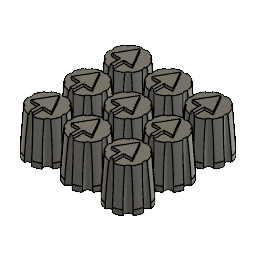
PotiKnobV3 (Autodesk Fusion 360 design; units mm, degrees)
Autodesk Fusion 360 part; units mm, degrees
sketch "Sketch1" plane through (0, 0, 0) normal (0, 1, 0) x (1, 0, 0)
  circle A0 centre (0, 0) radius 3.025
  circle A1 centre (0, 0) radius 7.5
  dimension "d1" = 6.05
  dimension "d2" = 15
  constraint coincident A0.centre A1.centre
  measures "d1" diameter of A0
  measures "d2" diameter of A1
extrude "Extrude1" add sketch "Sketch1" along normal blind 16 contours A0 | A1 makes body 1
extrude "Extrude2" cut sketch "Sketch1" along normal blind 12 contours A0 bodies 1
chamfer "Chamfer1" distance 1 distance2 3 1 edges at (-2.8203, 0, 1.0939) measured on face at (5.9804, 0, 0.3726) on bodies 1
sketch "Sketch2" plane through (0, 16, 0) normal (0, 1, 0) x (-1, 0, 0)
  circle A0 centre (0, 0) radius 7.5
  line L0 (0, 0) -> (0, -9.5957) construction
  circle A1 centre (0, -7.5) radius 1.3779
  circle A2 centre (5.3033, -5.3033) radius 1.3779
  circle A3 centre (7.5, 0) radius 1.3779
  circle A4 centre (5.3033, 5.3033) radius 1.3779
  circle A5 centre (0, 7.5) radius 1.3779
  circle A6 centre (-5.3033, 5.3033) radius 1.3779
  circle A7 centre (-7.5, 0) radius 1.3779
  circle A8 centre (-5.3033, -5.3033) radius 1.3779
  dimension "d10" = 360
  constraint coincident A0.centre L0.start
  constraint vertical L0
  constraint coincident L0 A1.centre
  constraint coincident A0 A1.centre
chamfer "Chamfer2" distance 1 distance2 14 1 edges at (-6.9925, 16, 2.7121) measured on face at (1.9158, 16, -2.8099) on bodies 1
extrude "Extrude3" cut sketch "Sketch2" against normal blind 17 contours A0 A3 | A0 A4 | A0 A2 | A0 A5 | A0 A1 | A0 A6 | A0 A8 | A0 A7 picked at (7.0559, -0.2871) picked at (4.9719, 4.9719) picked at (4.9719, -4.9719) picked at (0, 7.0313) picked at (0, -7.0313) picked at (-4.9932, 4.9519) picked at (-4.9932, -4.9519) picked at (-7.0313, 0) bodies 1
sketch "Sketch3" plane through (0, 16, 0) normal (0, 1, 0) x (-1, 0, 0)
  arc A0 (-3.9313, -5.1764) -> (-5.1764, -3.9313) centre (-5.3033, -5.3033) ccw
  arc A1 (-3.9313, -5.1764) -> (-0.8804, -6.4401) centre (0, 0) ccw
  arc A2 (0.8804, -6.4401) -> (-0.8804, -6.4401) centre (0, -7.5) ccw
  arc A3 (0.8804, -6.4401) -> (3.9313, -5.1764) centre (0, 0) ccw
  arc A4 (5.1764, -3.9313) -> (3.9313, -5.1764) centre (5.3033, -5.3033) ccw
  arc A5 (5.1764, -3.9313) -> (6.4401, -0.8804) centre (0, 0) ccw
  arc A6 (6.4401, 0.8804) -> (6.4401, -0.8804) centre (7.5, 0) ccw
  arc A7 (6.4401, 0.8804) -> (5.1764, 3.9313) centre (0, 0) ccw
  arc A8 (3.9313, 5.1764) -> (5.1764, 3.9313) centre (5.3033, 5.3033) ccw
  arc A9 (3.9313, 5.1764) -> (0.8804, 6.4401) centre (0, 0) ccw
  arc A10 (-0.8804, 6.4401) -> (0.8804, 6.4401) centre (0, 7.5) ccw
  arc A11 (-0.8804, 6.4401) -> (-3.9313, 5.1764) centre (0, 0) ccw
  arc A12 (-5.1764, 3.9313) -> (-3.9313, 5.1764) centre (-5.3033, 5.3033) ccw
  arc A13 (-5.1764, 3.9313) -> (-6.4401, 0.8804) centre (0, 0) ccw
  arc A14 (-6.4401, -0.8804) -> (-6.4401, 0.8804) centre (-7.5, 0) ccw
  arc A15 (-6.4401, -0.8804) -> (-5.1764, -3.9313) centre (0, 0) ccw
  line L0 (-4.0258, 2.3243) -> (0, -4.6486)
  line L1 (0, -4.6486) -> (4.0258, 2.3243)
  line L2 (4.0258, 2.3243) -> (-4.0258, 2.3243)
  line L3 (-0.6079, 6.7078) -> (0.6079, 6.7078)
  line L4 (0.6079, 6.7078) -> (0.6079, -6.7078)
  line L5 (0.6079, -6.7078) -> (-0.6079, -6.7078)
  line L6 (-0.6079, -6.7078) -> (-0.6079, 6.7078)
  line L7 (-0.6079, 6.7078) -> (0.6079, -6.7078) construction
  line L8 (0.6079, 6.7078) -> (-0.6079, -6.7078) construction
  constraint coincident A1.centre A3.centre
  constraint perpendicular L3 L4
  constraint parallel L3 L5
  constraint parallel L4 L6
  constraint horizontal L3
  constraint coincident L7 A1.centre
  constraint coincident L8 A1.centre
extrude "Extrude4" add sketch "Sketch3" along normal blind 1 contours L0 L1 L2 L4 L6 | L0 L2 L6 | L1 L2 L4 | A10 L2 L4 L6 bodies 1
pattern_linear "R-Pattern1" count 3 spacing 15.5 along (0, 0, 1) count 3 spacing 15.5 along (1, 0, 0) of bodies 1 makes body 2 at (3.0212, 9, 15.6508) makes body 3 at (3.0212, 9, 31.1508) makes body 4 at (18.5212, 9, 0.1508) makes body 5 at (18.5212, 9, 15.6508) makes body 6 at (18.5212, 9, 31.1508) makes body 7 at (34.0212, 9, 0.1508) makes body 8 at (34.0212, 9, 15.6508) makes body 9 at (34.0212, 9, 31.1508)
sketch "Sketch4" plane through (0, 0, 0) normal (0, 1, 0) x (1, 0, 0)
  line L0 (-12.5914, 11.0727) -> (43.6138, 11.0727)
  line L1 (43.6138, 11.0727) -> (43.6138, -43.6913)
  line L2 (43.6138, -43.6913) -> (-12.5914, -43.6913)
  line L3 (-12.5914, -43.6913) -> (-12.5914, 11.0727)
  constraint horizontal L0
  constraint vertical L1
  constraint horizontal L2
  constraint vertical L3
extrude "Extrude5" [suppressed]
